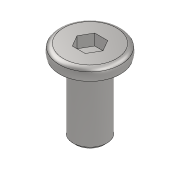
# Autodesk Inventor part: 10_051_LOW_HEAD_CAP_BOLT_M3X6_R1
Saved by Autodesk Inventor 2021.2 (Build 252289000, 289)
## iProperties
Created: 2020-05-03
Part Number: 10_051_LOW_HEAD_CAP_BOLT_M3X6_R1
Material: 一般
Document SubType Name: Modeling
Designer: y6tada
Density: 1 g/cm^3
Appearance: ステンレス - ブラシ仕上げ
Author: y6tada
Autodesk Inventor part; units mm, degrees
ref_plane "YZ Plane" through (0, 0, 0) normal (1, 0, 0) x (0, 1, 0)
ref_plane "XZ Plane" through (0, 0, 0) normal (0, 1, 0) x (-1, 0, 0)
ref_plane "XY Plane" through (0, 0, 0) normal (0, 0, 1) x (1, 0, 0)
sketch "スケッチ1" plane through (0, 0, 0) normal (0, 0, 1) x (1, 0, 0)
  line L0 (0, 0) -> (1.5, 0)
  line L1 (1.5, 0) -> (1.5, 6)
  line L2 (1.5, 6) -> (2.6, 6)
  line L3 (2.6, 6) -> (2.6, 7.2) construction
  line L4 (2.6, 7.2) -> (0, 7.2)
  line L5 (0, 7.2) -> (0, 0)
  line L6 (0, -5.542) -> (0, 0) construction
  arc A0 (2.6, 6) -> (2.6, 7.2) centre (1.8, 6.6) ccw
  line L7 (2.8, 9.0711) -> (2.8, 6.853) construction
  dimension "d0" = 3
  dimension "d1" = 6
  dimension "d2" = 5.2
  dimension "d3" = 1.2
  dimension "d13" = 5.6
  constraints: 16 end point, 5 perpendicular, 2 point on circle, 1 centre point, 1 collinear, 1 horizontal, 1 point on line, 1 tangent, 1 vertical
  measures "d0" diameter of L1 L6
  measures "d1" distance of L0.end L1.end
  measures "d2" diameter of L3 L6
  measures "d3" distance between parallel lines of L2 L4
  measures "d13" diameter of L7 L6
revolve "回転1" add sketch "スケッチ1" angle 360 about axis through (0, -5.542, 0) along (0, 1, 0)
sketch "スケッチ2" plane through (0, 7.2, 0) normal (0, 1, 0) x (1, 0, 0)
  line L0 (1.1547, 0) -> (0.5774, -1)
  line L1 (0.5774, -1) -> (-0.5774, -1)
  line L2 (-0.5774, -1) -> (-1.1547, 0)
  line L3 (-1.1547, 0) -> (-0.5774, 1)
  line L4 (-0.5774, 1) -> (0.5774, 1)
  line L5 (0.5774, 1) -> (1.1547, 0)
  line L6 (1.1547, 0) -> (-1.1547, 0) construction
  point P0 (0, 0)
  point P1 (0, 0)
  dimension "d5" = 2
  constraints: 14 end point, 1 coincident, 1 horizontal, 13 other
  measures "d5" distance between parallel lines of L1 L4
extrude "押し出し1" cut sketch "スケッチ2" against normal blind 1
fillet "フィレット1" radius 0.4 1 edges at (-2.6, 7.2, 0)
fillet "フィレット1" radius 0.3 1 edges at (-2.6, 6, 0)
chamfer "面取り1" distance 0.25 angle 45 1 edges at (-1.5, 0, 0)
